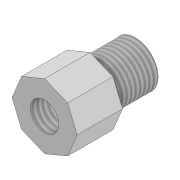
# Autodesk Inventor part: mark-10 adapter
Saved by Autodesk Inventor 2022 (Build 260153000, 153)
## iProperties
Created: 2022-06-16
Part Number: mark-10 adapter
Material: 일반
Document SubType Name: Modeling
Designer: Yeong Jae Park
Density: 1 g/cm^3
Appearance: 기본값
Author: Yeong Jae Park
Autodesk Inventor part; units mm, degrees
ref_plane "YZ Plane" through (0, 0, 0) normal (1, 0, 0) x (0, 1, 0)
ref_plane "XZ Plane" through (0, 0, 0) normal (0, 1, 0) x (-1, 0, 0)
ref_plane "XY Plane" through (0, 0, 0) normal (0, 0, 1) x (1, 0, 0)
sketch "스케치1" plane through (0, 0, 0) normal (0, 0, 1) x (1, 0, 0)
  circle A0 centre (0, 0) radius 6.35
  dimension "d0" = 12.7
  constraints: 1 centre point, 1 coincident
  measures "d0" diameter of A0
extrude "돌출1" add sketch "스케치1" along normal blind 10.16
sketch "스케치2" plane through (0, 0, 10.16) normal (0, 0, 1) x (1, 0, 0)
  circle A0 centre (0, 0) radius 6.35
  constraints: 1 centre point, 1 coincident
extrude "돌출2" add sketch "스케치2" along normal blind 15.24
thread "스레드1" size "1/2-20 UNF" class "2A" standard "ANSI Unified Screw Threads" length 12.7
sketch "스케치3" plane through (0, 0, 25.4) normal (0, 0, 1) x (1, 0, 0)
  circle A0 centre (0, 0) radius 3.9688
  dimension "d7" = 7.9375
  constraints: 1 centre point, 1 coincident
  measures "d7" diameter of A0
extrude "돌출3" cut sketch "스케치3" against normal blind 7.62
thread "스레드2" size "5/16-18 UNC" class "2B" standard "ANSI Unified Screw Threads" length 10.16
sketch "스케치4" plane through (0, 0, 25.4) normal (0, 0, 1) x (1, 0, 0)
  circle A0 centre (0, 0) radius 6.35 projected
  line L0 (0, 6.35) -> (0, -6.35) construction
  line L1 (-6.35, 0) -> (6.35, 0) construction
  line L2 (-6.35, 0) -> (-4.4901, 4.4901)
  line L3 (-4.4901, 4.4901) -> (0, 6.35)
  line L4 (0, 0) -> (-4.4901, 4.4901) construction
  line L5 (6.35, 0) -> (4.4901, 4.4901)
  line L6 (4.4901, 4.4901) -> (0, 6.35)
  line L7 (-6.35, 0) -> (-4.4901, -4.4901)
  line L8 (-4.4901, -4.4901) -> (0, -6.35)
  line L9 (4.4901, -4.4901) -> (0, -6.35)
  line L10 (6.35, 0) -> (4.4901, -4.4901)
  dimension "d12" = 45
  constraints: 22 end point, 5 point on circle, 4 midpoint, 3 symmetric about line, 1 horizontal, 1 vertical
  measures "d12" angle of L4 L1
extrude "돌출4" cut sketch "스케치4" against normal blind 12.7 contours L5 A0 | A0 L10 | L6 A0 | A0 L9 | L3 A0 | A0 L8 | L2 A0 | A0 L7
sketch "스케치5" plane through (0, 0, 25.4) normal (0, 0, 1) x (1, 0, 0)
  line L0 (4.4901, -4.4901) -> (6.35, 0) projected
  line L1 (6.35, 0) -> (4.4901, 4.4901) projected
  line L2 (4.4901, 4.4901) -> (0, 6.35) projected
  line L3 (0, 6.35) -> (-4.4901, 4.4901) projected
  line L4 (-4.4901, 4.4901) -> (-6.35, 0) projected
  line L5 (-6.35, 0) -> (-4.4901, -4.4901) projected
  line L6 (-4.4901, -4.4901) -> (0, -6.35) projected
  line L7 (0, -6.35) -> (4.4901, -4.4901) projected
  circle A0 centre (0, 0) radius 3.9687 projected
  line L8 (0, 9.0993) -> (6.4342, 6.4342)
  line L9 (6.4342, 6.4342) -> (9.0993, 0)
  line L10 (9.0993, 0) -> (6.4342, -6.4342)
  line L11 (6.4342, -6.4342) -> (0, -9.0993)
  line L12 (0, -9.0993) -> (-6.4342, -6.4342)
  line L13 (-6.4342, -6.4342) -> (-9.0993, 0)
  line L14 (-9.0993, 0) -> (-6.4342, 6.4342)
  line L15 (-6.4342, 6.4342) -> (0, 9.0993)
  dimension "d15" = 2.54
  constraints: 16 end point, 7 other
  measures "d15" distance between parallel lines of L2 L8
extrude "돌출5" add sketch "스케치5" against normal blind 12.7 contours L8 L9 L10 L11 L12 L13 L14 L15
